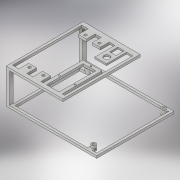
# Autodesk Inventor part: electronic_holder
Saved by Autodesk Inventor 2019 (Build 230136000, 136)
## iProperties
Created: 2020-05-07
Part Number: electronic_holder
Material: Generic
Document SubType Name: Modeling
Designer: Mateusz
Density: 1 g/cm^3
Appearance: Default
Author: Mateusz
Autodesk Inventor part; units mm, degrees
ref_plane "YZ Plane" through (0, 0, 0) normal (1, 0, 0) x (0, 1, 0)
ref_plane "XZ Plane" through (0, 0, 0) normal (0, 1, 0) x (-1, 0, 0)
ref_plane "XY Plane" through (0, 0, 0) normal (0, 0, 1) x (1, 0, 0)
sketch "Sketch1" plane through (0, 0, 0) normal (0, 1, 0) x (-1, 0, 0)
  circle A0 centre (0, 0) radius 1.65
  circle A1 centre (0, 0) radius 3
  circle A2 centre (5.12, 83.75) radius 1.65
  circle A3 centre (5.12, 83.75) radius 3
  circle A4 centre (93.53, 3.15) radius 1.65
  circle A5 centre (93.53, 3.15) radius 3
  line L0 (-6.58, 0) -> (-6.58, -6.22)
  line L1 (-6.58, -6.22) -> (-6.58, 91.53)
  line L2 (-6.58, 91.53) -> (103.15, 91.53)
  line L3 (103.15, 86.53) -> (103.15, -1.22)
  line L4 (103.15, -6.22) -> (-6.58, -6.22)
  line L5 (-6.58, 91.53) -> (-6.58, 88.53)
  line L6 (103.15, 91.53) -> (100.15, 91.53)
  line L7 (3, 0) -> (3, -3.22)
  line L8 (-3, 0) -> (-3, -3.22)
  line L9 (2.12, 83.75) -> (2.12, 88.53)
  line L10 (8.12, 83.75) -> (8.12, 88.53)
  line L11 (93.53, 6.15) -> (100.15, 6.15)
  line L12 (93.53, 0.15) -> (100.15, 0.15)
  line L13 (-3.58, 88.53) -> (-3.58, -3.22)
  line L14 (103.15, 91.53) -> (108.15, 91.53)
  line L15 (108.15, 91.53) -> (108.15, 86.53)
  line L16 (108.15, 86.53) -> (103.15, 86.53)
  line L17 (103.15, -6.22) -> (108.15, -6.22)
  line L18 (108.15, -6.22) -> (108.15, -1.22)
  line L19 (108.15, -1.22) -> (103.15, -1.22)
  line L20 (100.15, 88.53) -> (100.15, 6.15)
  line L21 (100.15, 0.15) -> (100.15, -3.22)
  line L22 (100.15, -3.22) -> (3, -3.22)
  line L23 (-3, -3.22) -> (-3.58, -3.22)
  line L24 (-3.58, 88.53) -> (2.12, 88.53)
  line L25 (8.12, 88.53) -> (100.15, 88.53)
  dimension "d0" = 3.3
  dimension "d1" = 6
  dimension "d4" = 3.3
  dimension "d5" = 6
  dimension "d8" = 3.3
  dimension "d9" = 6
  constraints: 52 end point, 25 perpendicular, 6 centre point, 6 point on circle, 6 tangent, 5 point on line, 4 coincident, 2 vertical
  measures "d0" diameter of A0
  measures "d1" diameter of A1
  measures "d4" diameter of A2
  measures "d5" diameter of A3
  measures "d8" diameter of A4
  measures "d9" diameter of A5
extrude "Extrusion1" add sketch "Sketch1" against normal blind 3 contours A1 | A5 | A3 | L1 L2 L14 L15 L16 L3 L19 L18 L17 L4 L0
extrude "Extrusion2" add sketch "Sketch1" along normal blind 3 contours A1 | A5 | A3
sketch "Sketch2" plane through (0, 0, 0) normal (0, 1, 0) x (1, 0, 0)
  line L0 (-103.15, 1.22) -> (-108.15, 1.22) projected
  line L1 (-103.15, 1.22) -> (-103.15, 6.22)
  line L2 (-108.15, 6.22) -> (6.58, 6.22) projected
  line L3 (-103.15, 6.22) -> (-108.15, 6.22)
  line L4 (-108.15, 6.22) -> (-108.15, 1.22)
  line L5 (-103.15, 1.22) -> (-103.15, -86.53) projected
  line L6 (-108.15, 1.22) -> (-103.15, 1.22)
  line L7 (-108.15, -91.53) -> (-108.15, -86.53) projected
  line L8 (-108.15, -91.53) -> (-103.15, -91.53)
  line L9 (6.58, -91.53) -> (-108.15, -91.53) projected
  line L10 (-103.15, -86.53) -> (-103.15, -91.53)
  line L11 (-108.15, -86.53) -> (-103.15, -86.53) projected
  line L12 (-103.15, -86.53) -> (-108.15, -86.53)
  line L13 (-108.15, -86.53) -> (-108.15, -91.53)
  line L14 (-103.15, -91.53) -> (-104.15, -91.53)
  line L15 (-104.15, -91.53) -> (-104.15, -86.53)
  line L16 (-103.15, 1.22) -> (-104.15, 1.22)
  line L17 (-104.15, 1.22) -> (-104.15, 6.22)
  point P0 (0, 0)
  dimension "d26" = 1
  dimension "d27" = 1
  constraints: 24 end point, 7 point on line, 5 perpendicular, 2 collinear, 1 vertical
  measures "d26" distance of L8.end L14.end
  measures "d27" distance of L0.start L16.end
extrude "Extrusion3" add sketch "Sketch2" along normal blind 41 contours L0 L4 L2 L17 | L15 L8 L7 L11
sketch "Sketch3" plane through (-104.15, 0, 91.53) normal (1, 0, 0) x (0, 0, -1)
  line L0 (0, 41) -> (5, 41) projected
  line L1 (0, 41) -> (0, 38)
  line L2 (0, -3) -> (0, 41) projected
  line L3 (0, 38) -> (5, 38)
  line L4 (5, -3) -> (5, 41) projected
  line L5 (5, 38) -> (5, 41)
  line L6 (5, 41) -> (0, 41)
  line L7 (92.75, 41) -> (97.75, 41) projected
  line L8 (92.75, 41) -> (92.75, 38)
  line L9 (92.75, -3) -> (92.75, 41) projected
  line L10 (92.75, 38) -> (97.75, 38)
  line L11 (97.75, -3) -> (97.75, 41) projected
  line L12 (97.75, 41) -> (92.75, 41)
  line L13 (97.75, 41) -> (97.75, 38)
  point P0 (91.53, 0)
  dimension "d30" = 3
  dimension "d31" = 3
  constraints: 16 end point, 5 point on line, 3 perpendicular, 1 vertical
  measures "d30" distance of L0.start L1.end
  measures "d31" distance of L7.start L8.end
extrude "Extrusion4" add sketch "Sketch3" along normal blind 35
sketch "Sketch4" plane through (0, 41, 0) normal (0, 1, 0) x (1, 0, 0)
  line L0 (-69.15, -91.53) -> (-69.15, -86.53) projected
  line L1 (-108.15, 1.22) -> (-69.15, 1.22) projected
  line L2 (-69.15, -86.53) -> (-69.15, -78.155)
  line L3 (-69.15, 1.22) -> (-69.15, -7.155)
  circle A0 centre (-74.23, -78.155) radius 1.65
  circle A1 centre (-74.23, -7.155) radius 1.65
  circle A2 centre (-92.01, -78.155) radius 1.65
  circle A3 centre (-92.01, -7.155) radius 1.65
  line L4 (-69.15, -78.155) -> (-69.15, -75.155)
  line L5 (-69.15, -75.155) -> (-69.15, -74.155)
  line L6 (-69.15, -74.155) -> (-97.09, -74.155)
  line L7 (-100.15, -88.53) -> (-100.15, -6.15) projected
  line L8 (-97.09, -74.155) -> (-97.09, -86.53)
  line L9 (-97.09, -86.53) -> (-69.15, -86.53)
  line L10 (-69.15, -7.155) -> (-69.15, -11.155)
  line L11 (-69.15, -11.155) -> (-97.09, -11.155)
  line L12 (-97.09, -11.155) -> (-97.09, 1.22)
  line L13 (-97.09, 1.22) -> (-69.15, 1.22)
  point P0 (0, 0)
  dimension "d46" = 3.3
  dimension "d47" = 3.3
  dimension "d50" = 3.3
  dimension "d51" = 3.3
  dimension "d53" = 1
  constraints: 22 end point, 6 perpendicular, 4 centre point, 4 point on line, 3 vertical
  measures "d46" diameter of A0
  measures "d47" diameter of A1
  measures "d50" diameter of A2
  measures "d51" diameter of A3
  measures "d53" distance of L4.end L5.end
extrude "Extrusion5" add sketch "Sketch4" against normal blind 3
sketch "Sketch5" plane through (-69.15, 0, 91.53) normal (1, 0, 0) x (0, 0, -1)
  line L0 (0, 41) -> (0, 38) projected
  line L1 (0, 41) -> (0, 38)
  line L2 (0, 41) -> (17.375, 41) projected
  line L3 (0, 41) -> (5, 41)
  line L4 (5, 41) -> (5, 38)
  line L5 (5, -3) -> (5, 41) projected
  line L6 (5, 38) -> (0, 38) projected
  line L7 (0, 38) -> (5, 38)
  line L8 (97.75, 38) -> (97.75, 41) projected
  line L9 (97.75, 41) -> (92.75, 41)
  line L10 (97.75, 41) -> (80.375, 41) projected
  line L11 (92.75, 38) -> (92.75, 41) projected
  line L12 (92.75, 41) -> (92.75, 38)
  line L13 (97.75, 38) -> (80.375, 38) projected
  line L14 (92.75, 38) -> (97.75, 38)
  line L15 (97.75, 38) -> (97.75, 41)
  point P0 (91.53, 0)
  dimension "d59" = 5
  dimension "d60" = 5
  constraints: 16 end point, 4 collinear, 3 point on line, 1 perpendicular
  measures "d59" distance of L0.start L3.end
  measures "d60" distance of L8.end L9.end
extrude "Extrusion6" add sketch "Sketch5" along normal blind 30
sketch "Sketch7" plane through (0, 41, 0) normal (0, 1, 0) x (1, 0, 0)
  line L0 (-69.15, 1.22) -> (-69.15, -11.155) projected
  line L1 (-69.15, 1.22) -> (-46.15, 1.22)
  line L2 (-3, 3.22) -> (-100.15, 3.22) projected
  line L3 (-69.15, 1.22) -> (-69.15, -11.155) projected
  line L4 (-69.15, -11.155) -> (-69.15, -25.405)
  line L5 (-69.15, -25.405) -> (-39.15, -25.405)
  line L6 (-39.15, 1.22) -> (-39.15, 6.22) projected
  line L7 (-39.15, -25.405) -> (-39.15, 1.22)
  line L8 (-39.15, 1.22) -> (-46.15, 1.22)
  circle A0 centre (-54.15, -17.905) radius 3.75
  point P0 (0, 0)
  dimension "d117" = 7.5
  constraints: 10 end point, 3 perpendicular, 1 centre point, 1 parallel, 1 point on line
  measures "d117" diameter of A0
extrude "Extrusion8" add sketch "Sketch7" against normal blind 2
sketch "Sketch8" plane through (0, 41, 0) normal (0, 1, 0) x (1, 0, 0)
  circle A0 centre (-74.23, -78.155) radius 1.65 projected
  circle A1 centre (-64.15, -68.155) radius 1
  circle A2 centre (-44.15, -68.155) radius 1
  circle A3 centre (-54.15, -38.155) radius 1
  line L0 (-39.15, -91.53) -> (-39.15, -86.53) projected
  line L1 (-39.15, -86.53) -> (-42.15, -86.53)
  line L2 (-42.15, -86.53) -> (-42.15, -39.155)
  line L3 (-42.15, -39.155) -> (-42.15, -36.155)
  line L4 (-66.15, -86.53) -> (-66.15, -36.155)
  line L5 (-66.15, -86.53) -> (-42.15, -86.53)
  line L6 (-66.15, -86.53) -> (-62.15, -86.53)
  line L7 (-69.15, -86.53) -> (-39.15, -86.53) projected
  line L8 (-42.15, -86.53) -> (-46.15, -86.53)
  line L9 (-62.15, -36.155) -> (-42.15, -36.155)
  line L10 (-62.15, -36.155) -> (-66.15, -36.155)
  line L11 (-46.15, -40.155) -> (-62.15, -40.155)
  line L12 (-62.15, -86.53) -> (-62.15, -40.155)
  line L13 (-46.15, -86.53) -> (-46.15, -40.155)
  point P0 (0, 0)
  dimension "d81" = 2
  dimension "d85" = 3
  dimension "d86" = 3
  dimension "d88" = 4
  dimension "d89" = 4
  constraints: 24 end point, 3 centre point, 3 perpendicular, 3 point on line, 1 parallel, 1 vertical
  measures "d81" diameter of A2
  measures "d85" distance of L0.end L1.end
  measures "d86" distance of L2.end L3.end
  measures "d88" distance of L4.start L6.end
  measures "d89" distance of L1.end L8.end
extrude "Extrusion9" add sketch "Sketch8" against normal blind 3 contours L5 L13 L11 L12 L4 L10 L9 L3 L2
sketch "Sketch9" plane through (0, 41, 0) normal (0, 1, 0) x (1, 0, 0)
  line L0 (-39.15, -91.53) -> (-36.15, -91.53)
  line L1 (-104.15, -91.53) -> (6.58, -91.53) projected
  line L2 (-36.15, -91.53) -> (-36.15, 6.22)
  line L3 (-108.15, 6.22) -> (6.58, 6.22) projected
  line L4 (-36.15, 6.22) -> (-39.15, 6.22)
  line L5 (-104.15, -91.53) -> (-39.15, -91.53) projected
  line L6 (-39.15, 6.22) -> (-39.15, -91.53)
  point P0 (0, 0)
  dimension "d94" = 3
  constraints: 8 end point, 2 perpendicular, 2 point on line, 1 horizontal
  measures "d94" distance of L0.start L0.end
extrude "Extrusion10" add sketch "Sketch9" against normal blind 3
sketch "Sketch10" plane through (0, 41, 0) normal (0, 1, 0) x (1, 0, 0)
  line L0 (-108.15, -86.53) -> (-103.15, -86.53) projected
  line L1 (-108.15, 6.22) -> (-108.15, 1.22) projected
  line L2 (-108.15, -86.53) -> (-108.15, 1.22)
  line L3 (-108.15, 1.22) -> (-105.15, 1.22)
  line L4 (-108.15, 1.22) -> (-97.09, 1.22) projected
  line L5 (-105.15, 1.22) -> (-105.15, -86.53)
  line L6 (-103.15, 1.22) -> (-103.15, -86.53) projected
  line L7 (-105.15, -86.53) -> (-108.15, -86.53)
  point P0 (0, 0)
  dimension "d97" = 3
  constraints: 8 end point, 1 parallel, 1 perpendicular, 1 point on line, 1 vertical
  measures "d97" distance of L1.end L3.end
extrude "Extrusion11" add sketch "Sketch10" against normal blind 3 contours L2 L3 L5 L0
sketch "Sketch11" plane through (0, 41, 0) normal (0, 1, 0) x (1, 0, 0)
  line L0 (-86.93, -78.155) -> (-86.93, -86.53)
  line L1 (-79.31, -78.155) -> (-79.31, -86.53)
  line L2 (-79.31, -86.53) -> (-86.93, -86.53)
  line L3 (-79.31, -78.155) -> (-79.31, -74.155)
  line L4 (-79.31, -74.155) -> (-86.93, -74.155)
  line L5 (-86.93, -78.155) -> (-86.93, -74.155)
  line L6 (-86.93, -7.155) -> (-86.93, 0)
  line L7 (-79.31, -7.155) -> (-79.31, 0)
  line L8 (-79.31, 0) -> (-86.93, 0)
  line L9 (-79.31, -7.155) -> (-79.31, -11.155)
  line L10 (-86.93, -7.155) -> (-86.93, -11.155)
  line L11 (-86.93, -11.155) -> (-79.31, -11.155)
  line L12 (-47.07, -17.905) -> (-47.07, 0)
  line L13 (-61.95, -17.905) -> (-61.95, 0)
  line L14 (-61.95, -17.905) -> (-61.95, -25.405)
  line L15 (-69.15, -25.405) -> (-39.15, -25.405) projected
  line L16 (-61.95, -25.405) -> (-47.07, -25.405)
  line L17 (-47.07, -25.405) -> (-47.07, -17.905)
  line L18 (-61.95, -25.405) -> (-69.15, -25.405)
  line L19 (-69.15, -25.405) -> (-69.15, 0)
  line L20 (-69.15, 1.22) -> (-69.15, -11.155) projected
  line L21 (-61.95, 0) -> (-69.15, 0)
  line L22 (-47.07, -25.405) -> (-39.15, -25.405)
  line L23 (-39.15, -25.405) -> (-39.15, 0)
  line L24 (-39.15, 0) -> (-47.07, 0)
  line L25 (-54.15, -17.905) -> (-54.15, -25.405)
  line L26 (-39.15, -25.405) -> (-69.15, -25.405) projected
  line L27 (-54.15, -25.405) -> (-54.15, -17.905)
  line L28 (-54.15, -17.905) -> (-54.15, -10.405)
  line L29 (-54.15, -10.405) -> (-58.15, -10.405)
  line L30 (-58.15, -10.405) -> (-58.15, 0)
  line L31 (-58.15, 0) -> (-50.15, 0)
  line L32 (-50.15, 0) -> (-50.15, -10.405)
  line L33 (-50.15, -10.405) -> (-54.15, -10.405)
  point P0 (0, 0)
  point P1 (-92.01, -78.155)
  point P2 (-74.23, -78.155)
  point P3 (-92.01, -7.155)
  dimension "d111" = 7.5
  dimension "d112" = 7.5
  dimension "d113" = 4
  dimension "d114" = 8
  constraints: 62 end point, 10 perpendicular, 6 point on line, 3 collinear, 1 horizontal, 1 midpoint, 1 vertical
  measures "d111" distance of L25.start L25.end
  measures "d112" distance of L25.start L28.end
  measures "d113" distance of L28.end L29.end
  measures "d114" distance of L30.end L31.end
extrude "Extrusion12" cut sketch "Sketch11" against normal blind 10
body "Solid1"
